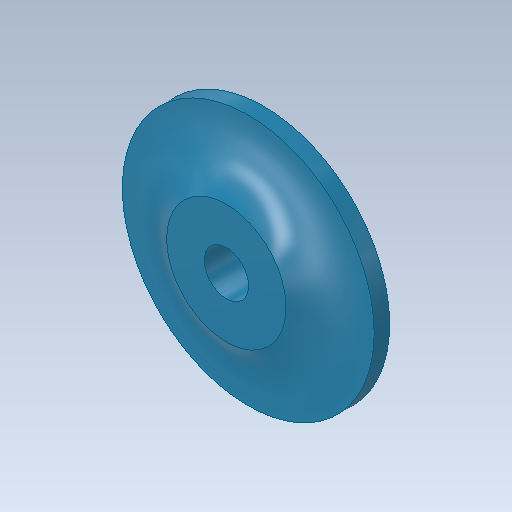
# Autodesk Inventor part: ダンパー１０
Saved by Autodesk Inventor 2020.2 (Build 242310000, 310)
## iProperties
Part Number: ダンパー１０
Material: アルミニウム 2014-T6
Document SubType Name: Modeling
Designer: suiky
Density: 2.78927 g/cm^3
Appearance: スカイ ブルー 濃い
Mass: 1.31058 g
Surface Area: 5.56055 cm^2
Volume: 0.469865 cm^3
Author: suiky
Autodesk Inventor part; units mm, degrees
ref_plane "YZ Plane" through (0, 0, 0) normal (1, 0, 0) x (0, 1, 0)
ref_plane "XZ Plane" through (0, 0, 0) normal (0, 1, 0) x (-1, 0, 0)
ref_plane "XY Plane" through (0, 0, 0) normal (0, 0, 1) x (1, 0, 0)
sketch "スケッチ1" plane through (0, 0, 0) normal (0, 0, 1) x (1, 0, 0)
  circle A0 centre (0, 0) radius 1.5
  circle A1 centre (0, 0) radius 8.5
  dimension "d0" = 3
  dimension "d1" = 17
  constraints: 2 centre point, 2 coincident
  measures "d0" diameter of A0
  measures "d1" diameter of A1
extrude "押し出し1" add sketch "スケッチ1" along normal blind 4
sketch "スケッチ2" plane through (0, 0, 0) normal (1, 0, 0) x (0, 1, 0)
  circle A0 centre (-8, 8.5) radius 6
  circle A1 centre (-8, -4.5) radius 6
  line L0 (-1.5, 4) -> (1.5, 4) projected
  line L1 (1.5, 0) -> (-1.5, 0) projected
  line L2 (-2, 12.4416) -> (-2, -10.3057) construction
  line L3 (-1.5, 0) -> (-1.5, 4) construction
  line L4 (-8, 8.5) -> (-8, -4.5) construction
  line L5 (-8, 8.5) -> (-8, 2) construction
  line L6 (-2, 4) -> (-2, 2)
  line L7 (-2, 4) -> (-2, -3)
  line L8 (8.5, 4) -> (-8.5, 4) projected
  line L9 (-1.5, 0) -> (-1.5, 4) projected
  line L10 (-2, 2) -> (-8, 2)
  point P0 (0, 0)
  dimension "d4" = 12
  dimension "d5" = 12
  dimension "d6" = 0.5
  dimension "d7" = 1
  dimension "d8" = 4
  dimension "d9" = 13
  dimension "d10" = 6.5
  dimension "d11" = 2
  dimension "d12" = 7
  constraints: 14 end point, 2 centre point, 2 collinear, 2 tangent, 1 horizontal, 1 midpoint, 1 point on line, 1 vertical
  measures "d4" diameter of A0
  measures "d5" diameter of A1
  measures "d6" distance between parallel lines of L2 L3
  measures "d8" distance of L1.end L0.start
  measures "d9" distance of L4.start L4.end
  measures "d10" distance of L4.start L5.end
  measures "d11" distance of L6.start L6.end
  measures "d12" distance of L6.start L7.end
sketch3d "3D スケッチ1"
  arc A0 (8.5, 0, 4) -> (0, 8.5, 4) centre (0, 0, 4) ccw
  arc A1 (0, 8.5, 4) -> (-8.5, 0, 4) centre (0, 0, 4) ccw
  arc A2 (-8.5, 0, 4) -> (0, -8.5, 4) centre (0, 0, 4) ccw
  arc A3 (0, -8.5, 4) -> (8.5, 0, 4) centre (0, 0, 4) ccw
sweep "スイープ1" cut profiles "スケッチ2" path "3D スケッチ1"
